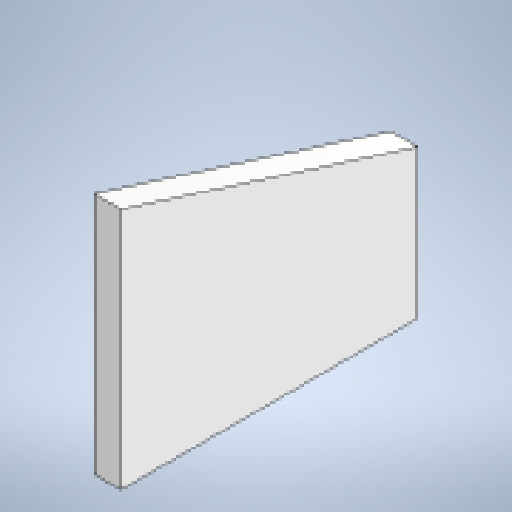
# Autodesk Inventor part: Front Plates
Saved by Autodesk Inventor 2023.2 (Build 272271000, 271)
## iProperties
Created: 2023-11-13
Part Number: Front Plates
Material: UHMW, White
Document SubType Name: Modeling
Designer: Nathan Cai
Density: 0.94 g/cm^3
Appearance: Smooth - White
Mass: 17.0585 g
Surface Area: 71.4408 cm^2
Volume: 18.1474 cm^3
Author: Nathan Cai
Autodesk Inventor part; units mm, degrees
ref_plane "YZ Plane" through (0, 0, 0) normal (1, 0, 0) x (0, 1, 0)
ref_plane "XZ Plane" through (0, 0, 0) normal (0, 1, 0) x (-1, 0, 0)
ref_plane "XY Plane" through (0, 0, 0) normal (0, 0, 1) x (1, 0, 0)
sketch "Sketch1" plane through (0, 0, 0) normal (1, 0, 0) x (0, 1, 0)
  line L0 (-17.4625, 34.925) -> (17.4625, 34.925)
  line L1 (17.4625, 34.925) -> (17.4625, -34.925)
  line L2 (17.4625, -34.925) -> (-17.4625, -34.925)
  line L3 (-17.4625, -34.925) -> (-17.4625, 34.925)
  line L4 (-17.4625, 34.925) -> (17.4625, -34.925) construction
  line L5 (17.4625, 34.925) -> (-17.4625, -34.925) construction
  line L6 (17.4625, -34.925) -> (39.6875, -34.925) construction
  line L7 (39.6875, -34.925) -> (39.6875, 34.925) construction
  line L8 (39.6875, 34.925) -> (17.4625, 34.925)
  line L9 (17.4625, 34.925) -> (17.4625, -34.925)
  line L10 (39.6875, 34.925) -> (17.4625, -34.925)
  point P0 (0, 0)
  dimension "d0" = 34.925
  dimension "d1" = 69.85
  dimension "d2" = 57.15
  constraints: 22 end point, 4 parallel, 2 horizontal, 2 midpoint, 2 perpendicular, 1 point on line
  measures "d0" distance of L1.end L2.end
  measures "d1" distance of L0.end L1.end
  measures "d2" distance between parallel lines of L3 L7
extrude "Extrusion1" add sketch "Sketch1" along normal blind 6.35
body "Solid1"
